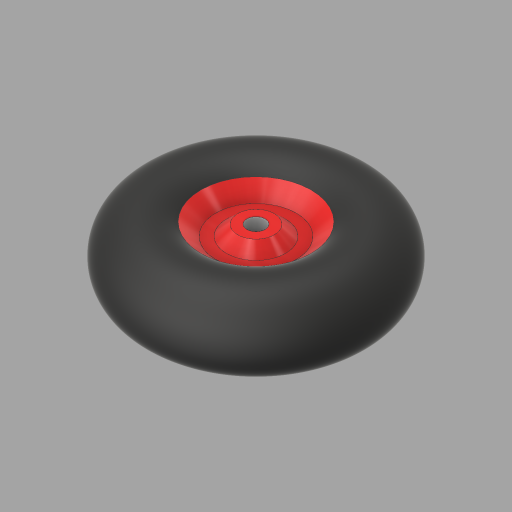
# Autodesk Inventor part: Wheel
Saved by Autodesk Inventor 2023.2 (Build 272271000, 271)
## iProperties
Created: 2023-02-01
Part Number: Wheel
Material: Generisch
Document SubType Name: Modeling
Designer: Raoul Messerli
Density: 1 g/cm^3
Appearance: Vorgabe
Author: Raoul Messerli
Autodesk Inventor part; units mm, degrees
ref_plane "YZ Plane" through (0, 0, 0) normal (1, 0, 0) x (0, 1, 0)
ref_plane "XZ Plane" through (0, 0, 0) normal (0, 1, 0) x (-1, 0, 0)
ref_plane "XY Plane" through (0, 0, 0) normal (0, 0, 1) x (1, 0, 0)
sketch "Skizze1" plane through (0, 0, 0) normal (1, 0, 0) x (0, 1, 0)
  line L0 (0, 0) -> (0, -60)
  line L1 (0, 0) -> (10, 0)
  line L2 (10, 0) -> (10, -60)
  line L3 (10, -60) -> (0, -60)
  line L4 (10, -60) -> (10, -60)
  line L5 (10, -60) -> (10, -8.2526)
  line L6 (10, -8.2526) -> (10, 0)
  line L7 (0, -30) -> (87.5, -30)
  circle A0 centre (87.5, -30) radius 42.5
  line L8 (10, 0) -> (20, 0)
  line L9 (10, -60) -> (20.0931, -60)
  line L10 (59.9602, 2.3699) -> (43.8038, -11.3757)
  line L11 (20, 0) -> (32.2885, -11.3757)
  line L12 (32.2885, -11.3757) -> (43.8038, -11.3757)
  line L13 (20.0931, -60) -> (32.2885, -48.6243)
  line L14 (32.2885, -48.6243) -> (43.8038, -48.6243)
  line L15 (43.8038, -48.6243) -> (59.9602, -62.3699)
  line L16 (38.0462, -11.3757) -> (38.0462, -48.6243)
  line L17 (130, -30) -> (87.5, -30)
  dimension "d0" = 20
  dimension "d1" = 60
  dimension "d2" = 85
  dimension "d4" = 260
  dimension "d5" = 40
  constraints: 36 end point, 6 horizontal, 4 point on circle, 3 midpoint, 3 perpendicular, 3 point on line, 3 vertical, 2 equal length, 2 tangent, 1 centre point, 1 coincident
  measures "d0" diameter of L2 L0
  measures "d1" distance of L0.start L0.end
  measures "d2" diameter of A0
  measures "d4" diameter of A0.start L0
  measures "d5" diameter of L8.end L0
revolve "Umdrehung1" add sketch "Skizze1" angle 360 about axis through (0, 0, 0) along (0, 0, -1) contours L8 L11 L12 L16 L7 L2 | L7 L16 L14 L13 L9 L2 | L16 L12 L10 A0 L7 | L7 A0 L15 L14 L16 | A0 L17 L7 | L7 L17 A0
